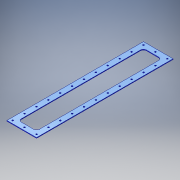
# Autodesk Inventor part: Gasket
Saved by Autodesk Inventor 2019.4 (Build 234330000, 330)
## iProperties
Created: 2020-04-27
Part Number: Gasket
Material: Generic
Document SubType Name: Modeling
Designer: Ed
Density: 1 g/cm^3
Appearance: Default
Author: Ed
Autodesk Inventor part; units mm, degrees
ref_plane "YZ Plane" through (0, 0, 0) normal (1, 0, 0) x (0, 1, 0)
ref_plane "XZ Plane" through (0, 0, 0) normal (0, 1, 0) x (-1, 0, 0)
ref_plane "XY Plane" through (0, 0, 0) normal (0, 0, 1) x (1, 0, 0)
sketch "Sketch1" plane through (0, 0, 0) normal (0, 1, 0) x (-1, 0, 0)
  line L0 (38.1, 44.45) -> (38.1, 277.8125)
  arc A0 (38.1, 44.45) -> (44.45, 38.1) centre (44.45, 44.45) ccw
  line L1 (72.39, 38.1) -> (44.45, 38.1)
  arc A1 (72.39, 38.1) -> (78.74, 44.45) centre (72.39, 44.45) ccw
  line L2 (78.74, 311.15) -> (78.74, 44.45)
  arc A2 (78.74, 311.15) -> (72.39, 317.5) centre (72.39, 311.15) ccw
  line L3 (44.45, 317.5) -> (72.39, 317.5)
  arc A3 (44.45, 317.5) -> (38.1, 311.15) centre (44.45, 311.15) ccw
  line L4 (38.1, 277.8125) -> (38.1, 311.15)
  arc A4 (31.4279, 295.675) -> (31.75, 295.6433) centre (31.75, 297.2943) ccw
  arc A5 (31.75, 295.6433) -> (33.401, 297.2943) centre (31.75, 297.2943) ccw
  arc A6 (33.401, 297.2943) -> (30.9245, 298.7241) centre (31.75, 297.2943) ccw
  arc A7 (30.9245, 298.7241) -> (30.3202, 298.1198) centre (31.75, 297.2943) ccw
  arc A8 (30.3202, 298.1198) -> (30.099, 297.2943) centre (31.75, 297.2943) ccw
  arc A9 (30.099, 297.2943) -> (31.4279, 295.675) centre (31.75, 297.2943) ccw
  arc A10 (31.3227, 269.1451) -> (33.401, 270.7399) centre (31.75, 270.7399) ccw
  arc A11 (33.401, 270.7399) -> (32.0721, 272.3591) centre (31.75, 270.7399) ccw
  arc A12 (32.0721, 272.3591) -> (31.3227, 272.3346) centre (31.75, 270.7399) ccw
  arc A13 (31.3227, 272.3346) -> (30.099, 270.7399) centre (31.75, 270.7399) ccw
  arc A14 (30.099, 270.7399) -> (31.3227, 269.1451) centre (31.75, 270.7399) ccw
  arc A15 (31.3227, 242.5907) -> (33.401, 244.1854) centre (31.75, 244.1854) ccw
  arc A16 (33.401, 244.1854) -> (31.3227, 245.7802) centre (31.75, 244.1854) ccw
  arc A17 (31.3227, 245.7802) -> (30.4402, 245.1905) centre (31.75, 244.1854) ccw
  arc A18 (30.4402, 245.1905) -> (30.099, 244.1854) centre (31.75, 244.1854) ccw
  arc A19 (30.099, 244.1854) -> (31.3227, 242.5907) centre (31.75, 244.1854) ccw
  arc A20 (31.3227, 216.0363) -> (33.401, 217.631) centre (31.75, 217.631) ccw
  arc A21 (33.401, 217.631) -> (32.0721, 219.2503) centre (31.75, 217.631) ccw
  arc A22 (32.0721, 219.2503) -> (31.3227, 219.2258) centre (31.75, 217.631) ccw
  arc A23 (31.3227, 219.2258) -> (30.099, 217.631) centre (31.75, 217.631) ccw
  arc A24 (30.099, 217.631) -> (31.3227, 216.0363) centre (31.75, 217.631) ccw
  arc A25 (31.3227, 189.4818) -> (33.401, 191.0766) centre (31.75, 191.0766) ccw
  arc A26 (33.401, 191.0766) -> (31.75, 192.7276) centre (31.75, 191.0766) ccw
  arc A27 (31.75, 192.7276) -> (30.5826, 192.244) centre (31.75, 191.0766) ccw
  arc A28 (30.5826, 192.244) -> (30.099, 191.0766) centre (31.75, 191.0766) ccw
  arc A29 (30.099, 191.0766) -> (31.3227, 189.4818) centre (31.75, 191.0766) ccw
  arc A30 (31.3227, 162.9274) -> (33.401, 164.5221) centre (31.75, 164.5221) ccw
  arc A31 (33.401, 164.5221) -> (32.0721, 166.1414) centre (31.75, 164.5221) ccw
  arc A32 (32.0721, 166.1414) -> (31.9923, 166.1553) centre (31.75, 164.5221) ccw
  arc A33 (31.9923, 166.1553) -> (31.75, 166.1731) centre (31.75, 164.5221) ccw
  arc A34 (31.75, 166.1731) -> (30.099, 164.5221) centre (31.75, 164.5221) ccw
  arc A35 (30.099, 164.5221) -> (31.3227, 162.9274) centre (31.75, 164.5221) ccw
  arc A36 (31.3227, 136.373) -> (33.401, 137.9677) centre (31.75, 137.9677) ccw
  arc A37 (33.401, 137.9677) -> (31.75, 139.6187) centre (31.75, 137.9677) ccw
  arc A38 (31.75, 139.6187) -> (30.5826, 139.1352) centre (31.75, 137.9677) ccw
  arc A39 (30.5826, 139.1352) -> (30.099, 137.9677) centre (31.75, 137.9677) ccw
  arc A40 (30.099, 137.9677) -> (31.3227, 136.373) centre (31.75, 137.9677) ccw
  arc A41 (31.3227, 109.8185) -> (33.401, 111.4133) centre (31.75, 111.4133) ccw
  arc A42 (33.401, 111.4133) -> (32.0721, 113.0326) centre (31.75, 111.4133) ccw
  arc A43 (32.0721, 113.0326) -> (31.9923, 113.0464) centre (31.75, 111.4133) ccw
  arc A44 (31.9923, 113.0464) -> (31.75, 113.0643) centre (31.75, 111.4133) ccw
  arc A45 (31.75, 113.0643) -> (30.099, 111.4133) centre (31.75, 111.4133) ccw
  arc A46 (30.099, 111.4133) -> (31.3227, 109.8185) centre (31.75, 111.4133) ccw
  arc A47 (31.3227, 83.2641) -> (33.401, 84.8589) centre (31.75, 84.8589) ccw
  arc A48 (33.401, 84.8589) -> (31.75, 86.5099) centre (31.75, 84.8589) ccw
  arc A49 (31.75, 86.5099) -> (30.8328, 86.2316) centre (31.75, 84.8589) ccw
  arc A50 (30.8328, 86.2316) -> (30.099, 84.8589) centre (31.75, 84.8589) ccw
  arc A51 (30.099, 84.8589) -> (31.3227, 83.2641) centre (31.75, 84.8589) ccw
  arc A52 (31.3227, 56.7097) -> (33.401, 58.3044) centre (31.75, 58.3044) ccw
  arc A53 (33.401, 58.3044) -> (32.0721, 59.9237) centre (31.75, 58.3044) ccw
  arc A54 (32.0721, 59.9237) -> (31.9923, 59.9376) centre (31.75, 58.3044) ccw
  arc A55 (31.9923, 59.9376) -> (31.75, 59.9554) centre (31.75, 58.3044) ccw
  arc A56 (31.75, 59.9554) -> (30.099, 58.3044) centre (31.75, 58.3044) ccw
  arc A57 (30.099, 58.3044) -> (31.3227, 56.7097) centre (31.75, 58.3044) ccw
  arc A58 (33.3447, 31.3227) -> (33.401, 31.75) centre (31.75, 31.75) ccw
  arc A59 (33.401, 31.75) -> (31.75, 33.401) centre (31.75, 31.75) ccw
  arc A60 (31.75, 33.401) -> (30.8328, 33.1228) centre (31.75, 31.75) ccw
  arc A61 (30.8328, 33.1228) -> (30.099, 31.75) centre (31.75, 31.75) ccw
  arc A62 (30.099, 31.75) -> (33.3447, 31.3227) centre (31.75, 31.75) ccw
  arc A63 (60.0569, 31.5345) -> (60.071, 31.75) centre (58.42, 31.75) ccw
  arc A64 (60.071, 31.75) -> (57.9927, 33.3447) centre (58.42, 31.75) ccw
  arc A65 (57.9927, 33.3447) -> (56.769, 31.75) centre (58.42, 31.75) ccw
  arc A66 (56.769, 31.75) -> (60.0147, 31.3227) centre (58.42, 31.75) ccw
  arc A67 (60.0147, 31.3227) -> (60.0569, 31.5345) centre (58.42, 31.75) ccw
  arc A68 (85.1305, 33.4005) -> (84.6627, 33.3447) centre (85.09, 31.75) ccw
  arc A69 (84.6627, 33.3447) -> (83.439, 31.75) centre (85.09, 31.75) ccw
  arc A70 (83.439, 31.75) -> (86.741, 31.75) centre (85.09, 31.75) ccw
  arc A71 (86.741, 31.75) -> (86.3662, 32.7974) centre (85.09, 31.75) ccw
  arc A72 (86.3662, 32.7974) -> (85.1305, 33.4005) centre (85.09, 31.75) ccw
  arc A73 (85.4121, 59.9237) -> (84.6627, 59.8992) centre (85.09, 58.3044) ccw
  arc A74 (84.6627, 59.8992) -> (83.439, 58.3044) centre (85.09, 58.3044) ccw
  arc A75 (83.439, 58.3044) -> (86.5198, 57.4789) centre (85.09, 58.3044) ccw
  arc A76 (86.5198, 57.4789) -> (86.741, 58.3044) centre (85.09, 58.3044) ccw
  arc A77 (86.741, 58.3044) -> (85.4121, 59.9237) centre (85.09, 58.3044) ccw
  arc A78 (85.1305, 86.5094) -> (84.6627, 86.4536) centre (85.09, 84.8589) ccw
  arc A79 (84.6627, 86.4536) -> (83.439, 84.8589) centre (85.09, 84.8589) ccw
  arc A80 (83.439, 84.8589) -> (84.6627, 83.2641) centre (85.09, 84.8589) ccw
  arc A81 (84.6627, 83.2641) -> (86.741, 84.8589) centre (85.09, 84.8589) ccw
  arc A82 (86.741, 84.8589) -> (86.3662, 85.9062) centre (85.09, 84.8589) ccw
  arc A83 (86.3662, 85.9062) -> (85.1305, 86.5094) centre (85.09, 84.8589) ccw
  arc A84 (85.4121, 113.0326) -> (84.6627, 113.008) centre (85.09, 111.4133) ccw
  arc A85 (84.6627, 113.008) -> (83.439, 111.4133) centre (85.09, 111.4133) ccw
  arc A86 (83.439, 111.4133) -> (86.5198, 110.5878) centre (85.09, 111.4133) ccw
  arc A87 (86.5198, 110.5878) -> (86.741, 111.4133) centre (85.09, 111.4133) ccw
  arc A88 (86.741, 111.4133) -> (85.4121, 113.0326) centre (85.09, 111.4133) ccw
  arc A89 (85.2249, 139.6132) -> (84.6627, 139.5625) centre (85.09, 137.9677) ccw
  arc A90 (84.6627, 139.5625) -> (83.439, 137.9677) centre (85.09, 137.9677) ccw
  arc A91 (83.439, 137.9677) -> (84.6627, 136.373) centre (85.09, 137.9677) ccw
  arc A92 (84.6627, 136.373) -> (86.741, 137.9677) centre (85.09, 137.9677) ccw
  arc A93 (86.741, 137.9677) -> (86.5707, 138.6979) centre (85.09, 137.9677) ccw
  arc A94 (86.5707, 138.6979) -> (85.2249, 139.6132) centre (85.09, 137.9677) ccw
  arc A95 (85.198, 166.1696) -> (84.2645, 165.952) centre (85.09, 164.5222) ccw
  arc A96 (84.2645, 165.952) -> (83.439, 164.5221) centre (85.09, 164.5222) ccw
  arc A97 (83.439, 164.5221) -> (86.2574, 163.3547) centre (85.09, 164.5222) ccw
  arc A98 (86.2574, 163.3547) -> (86.741, 164.5222) centre (85.09, 164.5222) ccw
  arc A99 (86.741, 164.5222) -> (85.5173, 166.1169) centre (85.09, 164.5222) ccw
  arc A100 (85.5173, 166.1169) -> (85.198, 166.1696) centre (85.09, 164.5222) ccw
  arc A101 (85.198, 192.724) -> (84.2645, 192.5064) centre (85.09, 191.0766) ccw
  arc A102 (84.2645, 192.5064) -> (83.439, 191.0766) centre (85.09, 191.0766) ccw
  arc A103 (83.439, 191.0766) -> (84.6627, 189.4818) centre (85.09, 191.0766) ccw
  arc A104 (84.6627, 189.4818) -> (86.741, 191.0766) centre (85.09, 191.0766) ccw
  arc A105 (86.741, 191.0766) -> (86.5198, 191.9021) centre (85.09, 191.0766) ccw
  arc A106 (86.5198, 191.9021) -> (85.198, 192.724) centre (85.09, 191.0766) ccw
  arc A107 (85.198, 219.2785) -> (84.2645, 219.0608) centre (85.09, 217.631) ccw
  arc A108 (84.2645, 219.0608) -> (83.439, 217.631) centre (85.09, 217.631) ccw
  arc A109 (83.439, 217.631) -> (86.2574, 216.4636) centre (85.09, 217.631) ccw
  arc A110 (86.2574, 216.4636) -> (86.741, 217.631) centre (85.09, 217.631) ccw
  arc A111 (86.741, 217.631) -> (85.5173, 219.2258) centre (85.09, 217.631) ccw
  arc A112 (85.5173, 219.2258) -> (85.198, 219.2785) centre (85.09, 217.631) ccw
  arc A113 (85.4912, 245.787) -> (83.9226, 245.3529) centre (85.09, 244.1854) ccw
  arc A114 (83.9226, 245.3529) -> (83.439, 244.1854) centre (85.09, 244.1854) ccw
  arc A115 (83.439, 244.1854) -> (84.6627, 242.5907) centre (85.09, 244.1854) ccw
  arc A116 (84.6627, 242.5907) -> (86.741, 244.1854) centre (85.09, 244.1854) ccw
  arc A117 (86.741, 244.1854) -> (86.6699, 244.6647) centre (85.09, 244.1854) ccw
  arc A118 (86.6699, 244.6647) -> (85.4912, 245.787) centre (85.09, 244.1854) ccw
  arc A119 (85.2518, 272.3829) -> (83.9226, 271.9073) centre (85.09, 270.7399) ccw
  arc A120 (83.9226, 271.9073) -> (83.439, 270.7399) centre (85.09, 270.7399) ccw
  arc A121 (83.439, 270.7399) -> (86.2574, 269.5724) centre (85.09, 270.7399) ccw
  arc A122 (86.2574, 269.5724) -> (86.741, 270.7399) centre (85.09, 270.7399) ccw
  arc A123 (86.741, 270.7399) -> (85.2518, 272.3829) centre (85.09, 270.7399) ccw
  arc A124 (85.5238, 298.8873) -> (83.4953, 297.7216) centre (85.09, 297.2943) ccw
  arc A125 (83.4953, 297.7216) -> (83.439, 297.2943) centre (85.09, 297.2943) ccw
  arc A126 (83.439, 297.2943) -> (84.6627, 295.6996) centre (85.09, 297.2943) ccw
  arc A127 (84.6627, 295.6996) -> (86.741, 297.2943) centre (85.09, 297.2943) ccw
  arc A128 (86.741, 297.2943) -> (86.6352, 297.8759) centre (85.09, 297.2943) ccw
  arc A129 (86.6352, 297.8759) -> (85.5238, 298.8873) centre (85.09, 297.2943) ccw
  arc A130 (83.4531, 324.0642) -> (83.439, 323.8487) centre (85.09, 323.8487) ccw
  arc A131 (83.439, 323.8487) -> (85.9155, 322.4189) centre (85.09, 323.8487) ccw
  arc A132 (85.9155, 322.4189) -> (86.741, 323.8487) centre (85.09, 323.8487) ccw
  arc A133 (86.741, 323.8487) -> (83.4953, 324.276) centre (85.09, 323.8487) ccw
  arc A134 (83.4953, 324.276) -> (83.4531, 324.0642) centre (85.09, 323.8487) ccw
  arc A135 (56.7831, 324.0655) -> (56.769, 323.85) centre (58.42, 323.85) ccw
  arc A136 (56.769, 323.85) -> (60.0147, 323.4227) centre (58.42, 323.85) ccw
  arc A137 (60.0147, 323.4227) -> (60.071, 323.85) centre (58.42, 323.85) ccw
  arc A138 (60.071, 323.85) -> (56.8253, 324.2773) centre (58.42, 323.85) ccw
  arc A139 (56.8253, 324.2773) -> (56.7831, 324.0655) centre (58.42, 323.85) ccw
  arc A140 (30.408, 324.8104) -> (30.1553, 324.276) centre (31.75, 323.8487) ccw
  arc A141 (30.1553, 324.276) -> (30.099, 323.8487) centre (31.75, 323.8487) ccw
  arc A142 (30.099, 323.8487) -> (30.5826, 322.6813) centre (31.75, 323.8487) ccw
  arc A143 (30.5826, 322.6813) -> (33.401, 323.8487) centre (31.75, 323.8487) ccw
  arc A144 (33.401, 323.8487) -> (30.408, 324.8104) centre (31.75, 323.8487) ccw
  line L5 (91.44, 330.2) -> (25.4, 330.2)
  line L6 (91.44, 25.4) -> (91.44, 330.2)
  line L7 (25.4, 25.4) -> (91.44, 25.4)
  line L8 (25.4, 330.2) -> (25.4, 25.4)
  point P0 (0, 0)
  constraints: 290 point on circle, 145 centre point, 28 equal radius, 18 end point, 8 tangent, 4 perpendicular, 3 parallel, 1 collinear
extrude "Extrusion1" add sketch "Sketch1" along normal blind 1.5875
body "Solid1"
